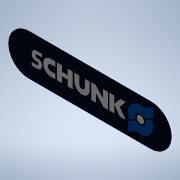
# Autodesk Inventor part: SCHUNK-9957615 Typenschild 16x64x0.3
Saved by Autodesk Inventor 2021 (Build 250183000, 183)
## iProperties
Created: 2025-07-30
Part Number: SCHUNK-9957615 Typenschild 16x64x0.3
Material: Generic
Catalog Web Link: www.cadenas.de
Description: Typenschild-SCHUNK-Typenschild
Vendor: SCHUNK
Document SubType Name: Modeling
Designer: psAdmin
Manufacturer: SCHUNK
Mass: 0.279207 g
Surface Area: 19.948 cm^2
Volume: 0.279207 cm^3
Density: 1 g/cm^3
Appearance: PSOLRGB-175-175-175
Category: PARTsolutions
Company: SCHUNK
Title: SCHUNK-9957615 Typenschild 16x64x0.3
Author: Cadenas PARTsolutions
Comments: SCHUNK-Typenschild
PSOL_IDENT_0: {$CADENAS_DATA/23d-libs/schunk/normteile/typenschilder.prj},217 {VTYP=3D},{NB=SCHUNK-9957615 Typensc
PSOL_IDENT_1: hild 16x64x0.3},{LINA=SCHUNK-9957615 Typenschild 16x64x0.3},{NN=Typenschild},{DATE=28.01.2025 09:52:
PSOL_IDENT_2: 53},{GEOMDATE=05.06.2024 07:11:39},{VERSION=},{LINEID=60},{WBVAR=},{WBNUMERIC=}  {NB=SCHUNK-9957615
PSOL_IDENT_3: Typenschild 16x64x0.3},{LINA=SCHUNK-9957615 Typenschild 16x64x0.3},{KT=DUMMY},{IDNR=9957615},{TYP=16
PSOL_IDENT_4: x64x0.3},{B=16.000},{L=64.000},{H=0.300},{SF=7.000},{SFL=5.900},{SFS=0.550},{SFBS=6.750},{VBS=1.150}
PSOL_IDENT_5: ,{VBC=0.900},{VBU=-1.250},{VL=20.000},{VS=-39.000},{TYP1=6.000},{PARTSERVER=1.000}
NB: SCHUNK-9957615 Typenschild 16x64x0.3
NN: Typenschild
NT: SCHUNK-Typenschild
NBSYN: SCHUNK-$IDNR. Typenschild $TYP.
LINA: SCHUNK-9957615 Typenschild 16x64x0.3
CATALOG: SCHUNK
IDNR: 9957615
TYP: 16x64x0.3
B: 16
L: 64
H: 0.3
SF: 7
SFL: 5.9
SFS: 0.55
SFBS: 6.75
VBS: 1.15
VBC: 0.9
VBU: -1.25
VL: 20
VS: -39
TYP1: 6
PARTSERVER: 1
SUPPLIER: SCHUNK
ARTICLENO: SCHUNK-9957615 Typenschild 16x64x0.3
BOMINFO: SCHUNK-9957615 Typenschild 16x64x0.3
CREATOR: CADENAS GmbH
Autodesk Inventor part; units mm, degrees
sketch "Sketch_1" plane through (0, 0, 0) normal (0, 0, 1) x (1, 0, 0)
  arc A0 (-32, 0) -> (-24, -8) centre (-24, 0) ccw
  line L0 (-24, -8) -> (24, -8)
  arc A1 (24, -8) -> (32, 0) centre (24, 0) ccw
  arc A2 (32, 0) -> (24, 8) centre (24, 0) ccw
  line L1 (24, 8) -> (-24, 8)
  arc A3 (-24, 8) -> (-32, 0) centre (-24, 0) ccw
  constraints: 8 point on circle, 4 centre point, 4 end point
extrude "Extrusion1" add sketch "Sketch_1" along normal blind 0.3
sketch "Sketch_13" plane through (0, 0, 0.3) normal (0, 0, 1) x (1, 0, 0)
  line L0 (-12.9184, 3.0554) -> (-12.9184, -3.0496)
  line L1 (-12.9184, -3.0496) -> (-10.8856, -3.0496)
  line L2 (-10.8856, -3.0496) -> (-10.8856, -0.7401)
  line L3 (-10.8856, -0.7401) -> (-8.6487, -0.7401)
  line L4 (-8.6487, -0.7401) -> (-8.6487, -3.0496)
  line L5 (-8.6487, -3.0496) -> (-6.6154, -3.0496)
  line L6 (-6.6154, -3.0496) -> (-6.6154, 3.0554)
  line L7 (-6.6154, 3.0554) -> (-8.6487, 3.0554)
  line L8 (-8.6487, 3.0554) -> (-8.6487, 0.8356)
  line L9 (-8.6487, 0.8356) -> (-10.8856, 0.8356)
  line L10 (-10.8856, 0.8356) -> (-10.8856, 3.0554)
  line L11 (-10.8856, 3.0554) -> (-12.9184, 3.0554)
  constraints: 24 end point
extrude "Extrusion2" cut sketch "Sketch_13" against normal blind 0.05
sketch "Sketch_15" plane through (0, 0, 0.3) normal (0, 0, 1) x (1, 0, 0)
  line L0 (0.5704, 3.0554) -> (0.5704, -3.0496)
  line L1 (0.5704, -3.0496) -> (2.5185, -3.0496)
  line L2 (2.5185, -3.0496) -> (2.5185, 0.0838)
  line L3 (2.5185, 0.0838) -> (5.4533, -3.0496)
  line L4 (5.4533, -3.0496) -> (7.188, -3.0496)
  line L5 (7.188, -3.0496) -> (7.188, 3.0554)
  line L6 (7.188, 3.0554) -> (5.2404, 3.0554)
  line L7 (5.2404, 3.0554) -> (5.2404, -0.0774)
  line L8 (5.2404, -0.0774) -> (2.3062, 3.0554)
  line L9 (2.3062, 3.0554) -> (0.5704, 3.0554)
  constraints: 20 end point
extrude "Extrusion3" cut sketch "Sketch_15" against normal blind 0.05
sketch "Sketch_16" plane through (0, 0, 0.3) normal (0, 0, 1) x (1, 0, 0)
  line L0 (7.711, 3.0554) -> (7.711, -3.0496)
  line L1 (7.711, -3.0496) -> (9.7438, -3.0496)
  line L2 (9.7438, -3.0496) -> (9.7438, -0.1709)
  line L3 (9.7438, -0.1709) -> (11.8624, -3.0496)
  line L4 (11.8624, -3.0496) -> (14.2863, -3.0496)
  line L5 (14.2863, -3.0496) -> (11.836, 0.2174)
  line L6 (11.836, 0.2174) -> (14.201, 3.0554)
  line L7 (14.201, 3.0554) -> (12.0659, 3.0554)
  line L8 (12.0659, 3.0554) -> (9.7438, 0.2895)
  line L9 (9.7438, 0.2895) -> (9.7438, 3.0554)
  line L10 (9.7438, 3.0554) -> (7.711, 3.0554)
  constraints: 22 end point
extrude "Extrusion4" cut sketch "Sketch_16" against normal blind 0.05
sketch "Sketch_5" plane through (0, 0, 0.3) normal (0, 0, 1) x (1, 0, 0)
  arc A0 (-22.8125, 0.7425) -> (-21.4625, -0.6075) centre (-21.4625, 0.7425) ccw
  line L0 (-21.4625, -0.6075) -> (-20.7538, -0.6075)
  arc A1 (-20.7538, -1.755) -> (-20.7538, -0.6075) centre (-20.7538, -1.1812) ccw
  line L1 (-20.7538, -1.755) -> (-22.8125, -1.755)
  line L2 (-22.8125, -1.755) -> (-22.8125, -3.0375)
  line L3 (-22.8125, -3.0375) -> (-20.6525, -3.0375)
  arc A2 (-20.6525, -3.0375) -> (-18.7625, -1.1475) centre (-20.6525, -1.1475) ccw
  line L4 (-18.7625, -1.1475) -> (-18.7625, -0.7425)
  arc A3 (-18.7625, -0.7425) -> (-20.1125, 0.6075) centre (-20.1125, -0.7425) ccw
  line L5 (-20.1125, 0.6075) -> (-20.7538, 0.6075)
  arc A4 (-20.7538, 1.755) -> (-20.7538, 0.6075) centre (-20.7358, 1.1812) ccw
  line L6 (-20.7538, 1.755) -> (-18.7625, 1.755)
  line L7 (-18.7625, 1.755) -> (-18.7625, 3.0375)
  line L8 (-18.7625, 3.0375) -> (-20.9225, 3.0375)
  arc A5 (-20.9225, 3.0375) -> (-22.8125, 1.1475) centre (-20.9225, 1.1475) ccw
  line L9 (-22.8125, 1.1475) -> (-22.8125, 0.7425)
  constraints: 20 end point, 12 point on circle, 6 centre point
extrude "Extrusion5" cut sketch "Sketch_5" against normal blind 0.05
sketch "Sketch_6" plane through (0, 0, 0.3) normal (0, 0, 1) x (1, 0, 0)
  arc A0 (-15.3, 3.0713) -> (-15.3, -3.0713) centre (-15.3, 0) ccw
  line L0 (-15.3, -3.0713) -> (-13.545, -3.0713)
  line L1 (-13.545, -3.0713) -> (-13.545, -1.1475)
  line L2 (-13.545, -1.1475) -> (-15.3, -1.1475)
  arc A1 (-15.3, 1.1475) -> (-15.3, -1.1475) centre (-15.3, 0) ccw
  line L3 (-15.3, 1.1475) -> (-13.545, 1.1475)
  line L4 (-13.545, 1.1475) -> (-13.545, 3.0713)
  line L5 (-13.545, 3.0713) -> (-15.3, 3.0713)
  constraints: 12 end point, 4 point on circle, 2 centre point
extrude "Extrusion6" cut sketch "Sketch_6" against normal blind 0.05
sketch "Sketch_7" plane through (0, 0, 0.3) normal (0, 0, 1) x (1, 0, 0)
  line L0 (-6.04, 2.97) -> (-6.04, 0)
  arc A0 (-6.04, 0) -> (0.035, 0) centre (-3.0025, 0) ccw
  line L1 (0.035, 0) -> (0.035, 2.97)
  line L2 (0.035, 2.97) -> (-1.9225, 2.97)
  line L3 (-1.9225, 2.97) -> (-1.9225, 0)
  arc A1 (-4.0825, 0) -> (-1.9225, 0) centre (-3.0025, 0) ccw
  line L4 (-4.0825, 0) -> (-4.0825, 2.97)
  line L5 (-4.0825, 2.97) -> (-6.04, 2.97)
  constraints: 12 end point, 4 point on circle, 2 centre point
extrude "Extrusion7" cut sketch "Sketch_7" against normal blind 0.05
sketch "Sketch8" plane through (0, 0, 0.3) normal (0, 0, 1) x (1, 0, 0)
  point P0 (20, 0)
hole "Hole1" at (20, 0, 0.3) direction (0, 0, -1) diameter 2.832 depth 0.05
sketch "Sketch_3" plane through (0, 0, 0.3) normal (0, 0, 1) x (1, 0, 0)
  arc A0 (21.4558, 4.7829) -> (15.4894, -2.1564) centre (20, 0) ccw
  line L0 (15.4894, -2.1564) -> (18.1798, -0.7416)
  arc A1 (21.6256, 1.1048) -> (18.1798, -0.7416) centre (20, 0) ccw
  line L1 (21.6256, 1.1048) -> (24.9442, 2.8689)
  line L2 (24.9442, 2.8689) -> (24.9442, 6.6331)
  line L3 (24.9442, 6.6331) -> (21.4558, 4.7829)
  constraints: 8 end point, 4 point on circle, 2 centre point
extrude "Extrusion8" cut sketch "Sketch_3" against normal blind 0.05
sketch "Sketch_4" plane through (0, 0, 0.3) normal (0, 0, 1) x (1, 0, 0)
  line L0 (15.0735, -2.8571) -> (15.0735, -6.6213)
  line L1 (15.0735, -6.6213) -> (18.5633, -4.7863)
  arc A0 (18.5633, -4.7863) -> (24.4981, 2.1771) centre (20, 0) ccw
  line L2 (24.4981, 2.1771) -> (21.8157, 0.7331)
  arc A1 (18.3864, -1.1091) -> (21.8157, 0.7331) centre (20, 0) ccw
  line L3 (18.3864, -1.1091) -> (15.0735, -2.8571)
  constraints: 8 end point, 4 point on circle, 2 centre point
extrude "Extrusion9" cut sketch "Sketch_4" against normal blind 0.05
ref_plane "aluschild_XY" through (0, 0, 0) normal (0, 0, 1) x (1, 0, 0)
ref_plane "aluschild_YZ" through (0, 0, 0) normal (1, 0, 0) x (0, 1, 0)
ref_plane "aluschild_ZX" through (0, 0, 0) normal (0, 1, 0) x (0, 0, 1)
body "Solid1"
